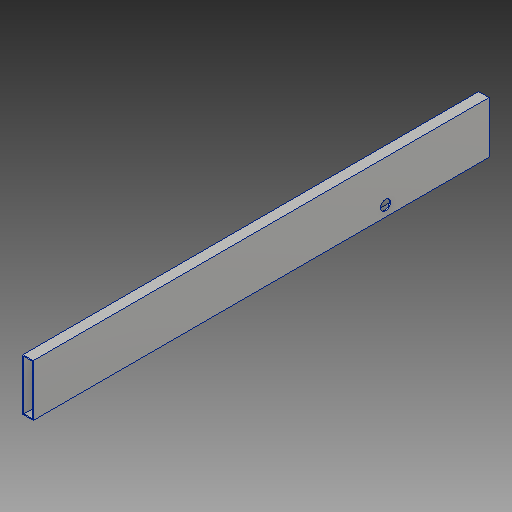
# Autodesk Inventor part: Side Extrusion
Saved by Autodesk Inventor 2019.4 (Build 234330000, 330)
## iProperties
Created: 2019-10-20
Part Number: Side Extrusion
Material: Aluminum 6061
Document SubType Name: Modeling
Designer: Mark
Density: 2.7 g/cm^3
Appearance: Aluminum - Flat
HoleDistanceX: 200.000 mm
Author: Mark
Autodesk Inventor part; units mm, degrees
ref_plane "YZ Plane" through (0, 0, 0) normal (1, 0, 0) x (0, 1, 0)
ref_plane "XZ Plane" through (0, 0, 0) normal (0, 1, 0) x (-1, 0, 0)
ref_plane "XY Plane" through (0, 0, 0) normal (0, 0, 1) x (1, 0, 0)
sketch "Sketch1" plane through (0, 0, 0) normal (0, 0, 1) x (1, 0, 0)
  line L0 (-10, -50) -> (10, -50)
  line L1 (10, -50) -> (10, 50)
  line L2 (10, 50) -> (-10, 50)
  line L3 (-10, 50) -> (-10, -50)
  line L4 (-10, -50) -> (10, 50) construction
  line L5 (10, -50) -> (-10, 50) construction
  line L6 (-8, -48) -> (8, -48)
  line L7 (8, -48) -> (8, 48)
  line L8 (8, 48) -> (-8, 48)
  line L9 (-8, 48) -> (-8, -48)
  line L10 (-8, -48) -> (8, 48) construction
  line L11 (8, -48) -> (-8, 48) construction
  point P0 (0, 0)
  dimension "d0" = 20
  dimension "d1" = 100
  dimension "d2" = 16
  dimension "d3" = 96
  constraints: 24 end point, 4 midpoint, 4 parallel, 2 horizontal, 2 perpendicular
  measures "d0" distance of L2.end L1.end
  measures "d1" distance of L1.end L0.end
  measures "d2" distance of L8.end L7.end
  measures "d3" distance of L7.end L6.end
extrude "Extrusion1" add sketch "Sketch1" along normal blind 880
sketch "Sketch2" plane through (-10, -50, 0) normal (-1, 0, 0) x (0, 0, 1)
  circle A0 centre (200, 20) radius 9.8
  line L0 (0, 100) -> (880, 100) projected
  line L1 (0, 100) -> (0, 0) projected
  point P0 (0, 50)
  dimension "d6" = 19.6
  dimension "d7" = 80
  dimension "HoleDistanceX" = 200
  constraints: 1 centre point
  measures "d6" diameter of A0
  measures "d7" distance from line of L0 A0.centre
  measures "HoleDistanceX" distance from line of L1 A0.centre
extrude "Extrusion2" cut sketch "Sketch2" against normal blind 880
equation "\"d7\" = Height"
equation "\"Height\" = 80"
body "Solid1"
